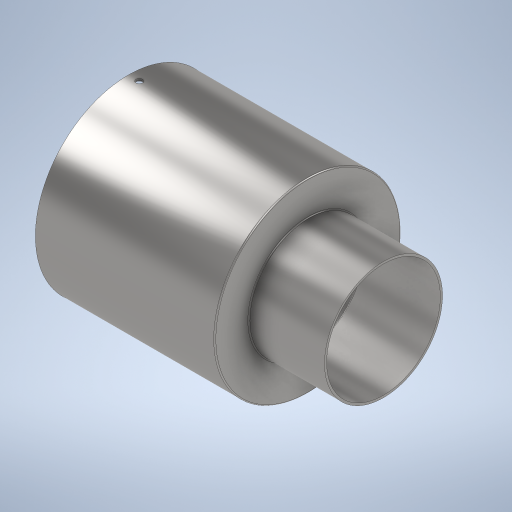
# Autodesk Inventor part: new outer wall
Saved by Autodesk Inventor 2023 (Build 270158000, 158)
## iProperties
Created: 2022-07-21
Part Number: new outer wall
Material: Stainless Steel
Document SubType Name: Modeling
Designer: station
Density: 8 g/cm^3
Appearance: Semi-Polished
Author: station
Autodesk Inventor part; units mm, degrees
ref_plane "YZ Plane" through (0, 0, 0) normal (1, 0, 0) x (0, 1, 0)
ref_plane "XY Plane" through (0, 0, 0) normal (0, 0, 1) x (1, 0, 0)
sketch "Sketch1" plane through (0, 0, 0) normal (0, 0, 1) x (1, 0, 0)
  line L0 (123.3912, 50.0622) -> (166.724, 25.044)
  line L1 (0, 3.5755) -> (319.1694, 3.5755)
  arc A0 (166.724, 25.044) -> (180.1312, 21.4516) centre (180.1312, 48.266) ccw
  arc A1 (180.0109, 21.4009) -> (182.0644, 21.7169) centre (180.0109, 28.2296) ccw
  line L2 (182.0644, 21.7169) -> (236.9947, 39.0364)
  arc A2 (123.3912, 50.0622) -> (30.0219, 75.0805) centre (30.0219, -111.6581) ccw
  line L3 (0, 75.0805) -> (30.0219, 75.0805)
  line L4 (180.1312, 33.0516) -> (237.115, 51.0185) construction
  line L5 (180.1312, 33.0516) -> (239.8803, 33.0516) construction
  line L6 (236.9947, 39.0364) -> (236.9947, 56.4) construction
  line L7 (180.1312, 33.0516) -> (180.1312, -12.2002)
  line L8 (180.0109, 33.433) -> (236.9947, 51.4)
  line L9 (236.9947, 51.4) -> (245.43, 54.0596)
  line L10 (166.724, 25.044) -> (166.724, 51.4) construction
  line L11 (166.724, 59.4) -> (166.724, 100.6805) construction
  line L12 (0, 88.1055) -> (30.0219, 88.1055)
  line L13 (30.0219, 88.1055) -> (162.724, 88.1055)
  line L14 (165.724, 90.1055) -> (30.0219, 90.1055)
  line L15 (30.0219, 90.1055) -> (0, 90.1055)
  line L16 (165.724, 90.1055) -> (165.724, 90.1055)
  line L17 (166.724, 89.1055) -> (166.724, 58.4)
  line L18 (164.724, 57.4) -> (164.724, 87.1055)
  line L19 (162.724, 88.1055) -> (163.724, 88.1055)
  line L20 (0, 88.1055) -> (0, 90.1055)
  line L21 (236.9947, 51.4) -> (236.9947, 53.4)
  arc A3 (164.724, 87.1055) -> (163.724, 88.1055) centre (163.724, 87.1055) ccw
  arc A4 (166.724, 89.1055) -> (165.724, 90.1055) centre (165.724, 89.1055) ccw
  line L22 (165.724, 56.4) -> (236.9947, 56.4)
  line L23 (167.724, 58.4) -> (236.9947, 58.4)
  line L24 (236.9947, 51.4) -> (236.9947, 58.4)
  arc A5 (164.724, 57.4) -> (165.724, 56.4) centre (165.724, 57.4) ccw
  arc A6 (166.724, 59.4) -> (167.724, 58.4) centre (167.724, 59.4) ccw
  point P0 (0, 0)
  point P1 (0, 0)
  point P2 (166.724, 88.6805)
  point P3 (166.724, 62.8622)
  point P4 (166.724, 90.1055)
  point P5 (164.724, 88.1055)
  dimension "d0" = 30.0219
  dimension "d1" = 186.7386
  dimension "d2" = 0
  dimension "d3" = 0
  dimension "d4" = 71.505
  dimension "d5" = 17.5
  dimension "d6" = 54.9303
  dimension "d8" = 17.5
  dimension "d15" = 0.4
  dimension "d23" = 13.025
  dimension "d24" = 2
  dimension "d28" = 2
  dimension "d32" = 1
  dimension "d45" = 2
  dimension "d46" = 1
  dimension "d47" = 17.3636
  constraints: 50 end point, 14 point on circle, 11 point on line, 8 tangent, 7 centre point, 5 horizontal, 4 parallel, 4 vertical, 3 perpendicular, 2 equal radius, 1 collinear, 1 equal length
  measures "d0" distance of L3.start L3.end
  measures "d1" radius of A2
  measures "d2" distance of A2.end L3.end
  measures "d3" distance of L0.start A2.start
  measures "d4" distance between parallel lines of L1 L3
  measures "d5" angle of L1 L2
  measures "d6" horizontal distance of L2.start L6.start
  measures "d8" angle of L5 L4
  measures "d15" distance between parallel lines of L4 L8
  measures "d23" distance between parallel lines of L3 L12
  measures "d24" distance between parallel lines of L13 L14
  measures "d28" distance between parallel lines of L11 L18
  measures "d32" radius of A3
  measures "d45" distance between parallel lines of L22 L23
  measures "d46" radius of A5
  measures "d47" distance of L6.start L6.end
revolve "Revolution3" add sketch "Sketch1" angle 360 about axis through (0, 3.5755, 0) along (1, 0, 0)
ref_plane "Work Plane1" through (0, 100, 0) normal (0, 1, 0) x (-1, 0, 0)
sketch "Sketch3" plane through (0, 100, 0) normal (0, 1, 0) x (-1, 0, 0)
  line L0 (0, 0) -> (-10, 0)
  circle A0 centre (-10, 0) radius 3
  dimension "d39" = 10
  dimension "d40" = 6
  constraints: 2 end point, 1 centre point, 1 coincident, 1 horizontal
  measures "d39" distance of L0.start L0.end
  measures "d40" diameter of A0
extrude "Extrusion2" cut sketch "Sketch3" against normal through all
thread "Thread1" size "M6x1" class "6H" standard "ANSI Metric M Profile" full length
body "Solid3"
